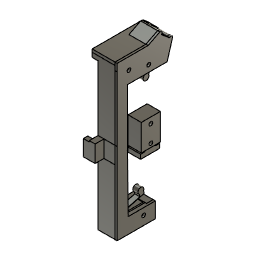
z_axis_switch v3 (Autodesk Fusion 360 design; units mm, degrees)
Autodesk Fusion 360 part; units mm, degrees
sketch "cnc " plane through (0, 0, 0) normal (1, 0, 0) x (0, 1, 0)
  line L0 (-75, 149.6) -> (-75, 72.1)
  line L1 (-75, 72.1) -> (-75, 61.1) construction
  line L2 (-75, 149.6) -> (-75, 160.6) construction
  line L3 (-75, 160.6) -> (-102, 160.6)
  line L4 (-102, 160.6) -> (-102, 61.1)
  line L5 (-102, 61.1) -> (-75, 61.1)
  line L6 (-75, 149.6) -> (-36, 149.6)
  line L7 (-75, 72.1) -> (-47, 72.1)
  line L8 (-47, 72.1) -> (-47, 61.1)
  line L9 (-47, 61.1) -> (-75, 61.1)
  line L10 (-75, 160.6) -> (-36, 160.6)
  line L11 (-36, 160.6) -> (-36, 149.6)
  line L12 (-75, 149.6) -> (-56, 149.6) construction
  line L13 (-56, 149.6) -> (-52, 149.6) construction
  line L14 (-52, 149.6) -> (-60, 149.6) construction
  line L15 (-60, 149.6) -> (-60, 67) construction
  line L16 (-60, 67) -> (-52, 67) construction
  line L17 (-52, 67) -> (-52, 149.6) construction
  line L18 (-8.6261, 128.7317) -> (-68.6261, 128.7317)
  line L19 (-68.6261, 128.7317) -> (-68.6261, 94.7317)
  line L20 (-68.6261, 94.7317) -> (-8.6261, 94.7317)
  line L21 (-8.6261, 94.7317) -> (-8.6261, 128.7317)
  dimension "d1" = 77.5
  dimension "d2" = 11
  dimension "d3" = 11
  dimension "d4" = 27
  dimension "d5" = 39
  dimension "d6" = 28
  dimension "d7" = 19
  dimension "d9" = 8
  dimension "d10" = 60
  dimension "d11" = 34
  constraint vertical L0
  constraint parallel L0 L1
  constraint vertical L2
  constraint perpendicular L2 L3
  constraint perpendicular L3 L4
  constraint perpendicular L1 L5
  constraint perpendicular L2 L6
  constraint perpendicular L1 L7
  constraint perpendicular L5 L8
  constraint perpendicular L8 L9
  constraint perpendicular L2 L10
  constraint perpendicular L6 L11
  constraint perpendicular L0 L12
  constraint parallel L6 L13
  constraint horizontal L14
  constraint vertical L15
  constraint horizontal L16
  constraint vertical L17
  constraint horizontal L18
  constraint vertical L19
  constraint horizontal L20
  constraint vertical L21
  measures "d1" distance of L0.start L0.end
  measures "d2" distance of L0.end L1.end
  measures "d3" distance of L0.start L2.end
  measures "d4" distance of L2.end L3.end
  measures "d5" distance of L0.start L6.end
  measures "d6" distance of L0.end L7.end
  measures "d7" distance of L0.start L12.end
  measures "d9" distance of L13.end L14.end
  measures "d10" distance of L18.start L18.end
  measures "d11" distance of L18.start L20.end
sketch "bracket base" plane through (0, 0, 0) normal (1, 0, 0) x (0, 1, 0)
  line L0 (-75, 111.25) -> (-88, 111.25) construction
  line L1 (-75, 111.25) -> (-77, 111.25) construction
  line L2 (-77, 111.25) -> (-77, 105.5) construction
  line L3 (-77, 105.5) -> (-80, 105.5)
  line L4 (-80, 105.5) -> (-80, 116.25)
  line L5 (-80, 116.25) -> (-77, 116.25)
  line L6 (-77, 116.25) -> (-77, 105.5)
  line L7 (-80, 117) -> (-74, 117)
  line L8 (-74, 117) -> (-74, 105.5)
  line L9 (-74, 105.5) -> (-80, 105.5)
  line L10 (-80, 105.5) -> (-80, 117)
  line L11 (-74, 161) -> (-74, 117)
  line L12 (-67, 149.9652) -> (-67, 111.25)
  line L13 (-48.0004, 72.0159) -> (-48.0011, 61.5)
  line L14 (-67, 72.0348) -> (-67, 111.25)
  line L15 (-74, 61.5) -> (-74, 105.5)
  line L16 (-74, 61.5) -> (-48.0011, 61.5)
  circle A0 centre (-56, 67.5) radius 1.25
  circle A1 centre (-66, 158) radius 1.25
  line L17 (-67, 149.9652) -> (-40.0004, 149.992)
  line L18 (-74, 161) -> (-74, 164.0222)
  line L19 (-74, 164.0222) -> (-40.0011, 163.9932)
  line L20 (-67, 72.0348) -> (-48.0004, 72.0159)
  circle A2 centre (-52.5121, 154.5) radius 1.25
  circle A3 centre (-59.5121, 154.5) radius 0.9
  circle A4 centre (-63, 67.5) radius 0.9
  line L21 (-68.5, 152) -> (-68.5, 69.9959)
  line L22 (-66, 66) -> (-66, 72)
  line L23 (-53, 72) -> (-53, 66)
  line L24 (-62.5121, 155.9825) -> (-62.5121, 149.9825)
  line L25 (-49.5121, 149.9825) -> (-49.5121, 155.9825)
  line L26 (-68.5, 152) -> (-63.083, 152)
  line L27 (-63.083, 152) -> (-63.081, 149.9691)
  line L28 (-68.5, 69.9959) -> (-66.5, 69.9959)
  line L29 (-66.5, 69.9959) -> (-66.5, 72.0343)
  line L30 (-72.5, 164.0209) -> (-72.5, 61.5)
  line L31 (-49, 152) -> (-48.998, 149.9831)
  line L32 (-49, 152) -> (-42.0325, 152.0069)
  line L33 (-57.0005, 161) -> (-57.0005, 164.0077)
  line L34 (-57.0005, 164.0077) -> (-45, 170)
  line L35 (-36.3287, 162.5038) -> (-40.0004, 149.992)
  line L36 (-40.0011, 163.9932) -> (-36.3, 163.9932)
  line L37 (-38.345, 163.1699) -> (-42.0325, 152.0069)
  line L38 (-57.0005, 161) -> (-43.8745, 167.8402)
  arc A5 (-43.8745, 167.8402) -> (-45, 170) centre (-44.7427, 168.7609) ccw
  arc A6 (-36.3287, 162.5038) -> (-38.345, 163.1699) centre (-37.3657, 162.7495) ccw
  line L39 (-43.6205, 169.3458) -> (-36.6837, 163.5684)
  line L40 (-40.0011, 161) -> (-36.77, 161)
  line L41 (-40.0011, 161) -> (-74, 161)
  line L42 (-47, 62.5) -> (-72.5, 62.5)
  line L43 (-50, 72.5) -> (-50, 62.5)
  line L44 (-52.5, 72.5) -> (-52.5, 69.9959)
  line L45 (-52.5, 69.9959) -> (-50, 69.9959)
  line L46 (-74, 166) -> (-40.1038, 166)
  line L47 (-74, 164.0222) -> (-74, 166)
  circle A7 centre (-45, 155) radius 1.25
  circle A8 centre (-43, 162) radius 1.25
  circle A9 centre (-66, 158) radius 3
  line L48 (-46.25, 155.0105) -> (-48.5, 159.5)
  line L49 (-46.524, 160.4903) -> (-43.7645, 155.19)
  arc A10 (-46.524, 160.4903) -> (-48.5, 159.5) centre (-47.5044, 159.9799) ccw
  line L50 (-40.1038, 166) -> (-39.6033, 166)
  circle A11 centre (-67.75, 66.5) radius 1.25
  dimension "d46" = 2.5
  dimension "d47" = 2.5
  dimension "d99" = 2.5
  dimension "d100" = 1.8
  dimension "d101" = 1.8
  dimension "d135" = 13
  dimension "d136" = 6
  dimension "d139" = 2.5
  dimension "d140" = 2.5
  dimension "d141" = 2.5
  constraint coincident L0 L1.end
  constraint perpendicular L0 L2
  constraint horizontal L3
  constraint vertical L4
  constraint horizontal L5
  constraint vertical L6
  constraint horizontal L7
  constraint vertical L8
  constraint horizontal L9
  constraint vertical L10
  constraint perpendicular L0 L12
  constraint coincident L16 L30.end
  constraint perpendicular L21 L26
  constraint coincident L17 L27.end
  constraint perpendicular L17 L27
  constraint perpendicular L22 L28
  constraint coincident L20 L29.end
  constraint perpendicular L28 L29
  constraint coincident L19 L30.start
  constraint coincident L17 L31.end
  constraint perpendicular L17 L31
  constraint perpendicular L31 L32
  constraint midpoint L19 L33.end
  constraint vertical L33
  constraint horizontal L36
  constraint midpoint A5 L39.start
  constraint coincident A6 L39.end
  constraint tangent A6 L39
  constraint coincident L35 L40.end
  constraint coincident L30 L42.end
  constraint perpendicular L30 L42
  constraint coincident L42 L43.end
  constraint perpendicular L42 L43
  constraint perpendicular L28 L44
  constraint coincident L43 L45.end
  constraint perpendicular L43 L45
  constraint perpendicular L46 L47
  constraint concentric A1 A9
  constraint coincident A7 L48.start
  constraint coincident A7 L49.end
  constraint tangent L49 A10
  constraint coincident L39 L50.end
  constraint parallel L46 L50
  measures "d46" diameter of A0
  measures "d47" diameter of A1
  measures "d99" diameter of A2
  measures "d100" diameter of A3
  measures "d101" diameter of A4
  measures "d135" distance of L25.start L24.end
  measures "d136" distance of L24.start L24.end
  measures "d139" diameter of A7
  measures "d140" diameter of A8
  measures "d141" diameter of A11
sketch "switches" plane through (0, 0, 0) normal (1, 0, 0) x (0, 1, 0)
  line L0 (0, 2.5) -> (0, 20)
  line L1 (-53, 66) -> (-66, 66)
  line L2 (-64.544, 66) -> (-64.544, 63)
  line L3 (-59.244, 66) -> (-59.244, 63)
  arc A0 (-51.9175, 78.8916) -> (-54.8153, 78.1152) centre (-53.3664, 78.5034) ccw
  line L4 (-51.141, 75.9939) -> (-51.0745, 75.7529)
  line L5 (-55, 65.5) -> (-54.514, 66)
  line L6 (-54.514, 63) -> (-54.514, 66)
  line L7 (-66, 66) -> (-66, 72)
  circle A1 centre (-53.3664, 78.5034) radius 2
  circle A2 centre (-56, 67.5) radius 0.9
  line L8 (-54.014, 66) -> (-54.014, 63)
  line L9 (-59.244, 63) -> (-59.744, 63)
  line L10 (-65.0804, 72) -> (-65.1451, 72.2415)
  line L11 (-64, 65.5) -> (-62, 65.5)
  line L12 (-57, 65.5) -> (-55, 65.5)
  line L13 (-54.0388, 75.2174) -> (-54.8153, 78.1152)
  line L14 (-65.044, 63) -> (-65.044, 66)
  line L15 (-66, 72) -> (-53, 72)
  circle A3 centre (-63, 67.5) radius 0.9
  line L16 (-51.141, 75.9939) -> (-51.9175, 78.8916)
  line L17 (-64, 65.5) -> (-64.5144, 66)
  line L18 (-51.141, 75.9939) -> (-54.0388, 75.2174)
  line L19 (-65.1451, 72.2415) -> (-51.141, 75.9939)
  line L20 (-65.0804, 72) -> (-51.0745, 75.7529)
  line L21 (-59.744, 66) -> (-59.244, 66)
  line L22 (-54.514, 66) -> (-54.014, 66)
  line L23 (-65.044, 66) -> (-64.544, 66)
  line L24 (-59.744, 63) -> (-59.744, 66)
  line L25 (-64.544, 63) -> (-65.044, 63)
  line L26 (-53, 72) -> (-53, 66)
  line L27 (-62, 65.5) -> (-61.514, 66)
  line L28 (-54.014, 63) -> (-54.514, 63)
  line L29 (-57, 65.5) -> (-57.5144, 66)
  line L30 (-47.6531, 145.9886) -> (-50.5509, 146.7651)
  line L31 (-61.6572, 149.741) -> (-47.6531, 145.9886)
  line L32 (-51.026, 155.9825) -> (-50.526, 155.9825)
  line L33 (-60.5121, 156.4825) -> (-58.5121, 156.4825)
  line L34 (-50.5509, 146.7651) -> (-51.3273, 143.8673)
  line L35 (-49.5121, 149.9825) -> (-49.5121, 155.9825)
  circle A4 centre (-49.8784, 143.4791) radius 2
  line L36 (-51.026, 158.9825) -> (-51.026, 155.9825)
  line L37 (-61.056, 155.9825) -> (-61.056, 158.9825)
  line L38 (-53.5121, 156.4825) -> (-54.0264, 155.9825)
  line L39 (-50.526, 158.9825) -> (-51.026, 158.9825)
  line L40 (-61.5925, 149.9825) -> (-47.5865, 146.2296)
  line L41 (-56.256, 158.9825) -> (-56.256, 155.9825)
  line L42 (-61.5925, 149.9825) -> (-61.6572, 149.741)
  line L43 (-62.5121, 155.9825) -> (-62.5121, 149.9825)
  line L44 (-53.5121, 156.4825) -> (-51.5121, 156.4825)
  line L45 (-47.6531, 145.9886) -> (-47.5865, 146.2296)
  line L46 (-51.5121, 156.4825) -> (-51.026, 155.9825)
  line L47 (-56.256, 155.9825) -> (-55.756, 155.9825)
  line L48 (-61.056, 158.9825) -> (-61.556, 158.9825)
  circle A5 centre (-52.5121, 154.4825) radius 0.9
  arc A6 (-51.3273, 143.8673) -> (-48.4296, 143.0909) centre (-49.8784, 143.4791) ccw
  circle A7 centre (-59.5121, 154.4825) radius 0.9
  line L49 (-61.556, 155.9825) -> (-61.056, 155.9825)
  line L50 (-58.5121, 156.4825) -> (-58.026, 155.9825)
  line L51 (-62.5121, 149.9825) -> (-49.5121, 149.9825)
  line L52 (-55.756, 155.9825) -> (-55.756, 158.9825)
  line L53 (-50.526, 155.9825) -> (-50.526, 158.9825)
  line L54 (-47.6531, 145.9886) -> (-48.4296, 143.0909)
  line L55 (-60.5121, 156.4825) -> (-61.0264, 155.9825)
  line L56 (-49.5121, 155.9825) -> (-62.5121, 155.9825)
  line L57 (-55.756, 158.9825) -> (-56.256, 158.9825)
  line L58 (-61.556, 158.9825) -> (-61.556, 155.9825)
  line L59 (-57.6, 101) -> (-44.6, 101)
  line L60 (-57.6, 123) -> (-44.6, 123)
  line L61 (-57.6, 123) -> (-57.6, 105)
  line L62 (-57.6, 105) -> (-44.6, 105)
  line L63 (-44.6, 105) -> (-44.6, 123)
  circle A8 centre (-51.1, 119) radius 1.25
  circle A9 centre (-51.1, 107.5) radius 1.25
  line L64 (-44.6, 101) -> (-44.6, 104)
  line L65 (-44.6, 104) -> (-47.6, 104)
  line L66 (-47.6, 104) -> (-47.6, 121)
  line L67 (-47.6, 121) -> (-54.6, 121)
  line L68 (-54.6, 121) -> (-54.6, 105)
  line L69 (-57.6, 101) -> (-57.6, 104)
  line L70 (-57.6, 104) -> (-54.6, 104)
  line L71 (-54.6, 104) -> (-54.6, 105)
  line L72 (-52.3542, 105) -> (-52.3542, 121)
  line L73 (-49.8734, 105) -> (-49.8734, 121)
  line L74 (-49.8784, 143.4791) -> (-49.8784, 65) construction
  line L75 (-53.3664, 78.5034) -> (-53.3664, 167.4772) construction
  dimension "d74" = 13
  dimension "d75" = 6
  dimension "d76" = 1.8
  dimension "d77" = 1.8
  dimension "d78" = 0.5
  dimension "d79" = 3
  dimension "d80" = 0.5
  dimension "d81" = 3
  dimension "d82" = 0.5
  dimension "d83" = 3
  dimension "d85" = 14.5
  dimension "d86" = 0.25
  dimension "d87" = 3
  dimension "d88" = 3
  dimension "d89" = 3
  dimension "d90" = 4
  dimension "d91" = 2.5
  dimension "d92" = 2.5
  dimension "d97" = 1.8
  dimension "d98" = 1.8
  constraint coincident L50.end L56
  constraint coincident L55.end L56
  constraint perpendicular L50 L55
  constraint parallel L44 L56
  constraint coincident L32.start L56
  constraint parallel L46 L50
  constraint coincident L38.end L56
  constraint perpendicular L38 L50
  constraint coincident L40.start L51
  constraint perpendicular L40 L42
  constraint perpendicular L31 L42
  constraint perpendicular L31 L54
  constraint perpendicular L30 L54
  constraint perpendicular L31 L34
  constraint tangent A6 L54
  constraint concentric A4 A6
  constraint horizontal L59
  constraint horizontal L60
  constraint perpendicular L60 L61
  constraint perpendicular L61 L62
  constraint perpendicular L60 L63
  constraint perpendicular L59 L64
  constraint perpendicular L64 L65
  constraint perpendicular L60 L66
  constraint perpendicular L66 L67
  constraint coincident L62 L68.end
  constraint perpendicular L60 L68
  constraint perpendicular L59 L69
  constraint perpendicular L69 L70
  constraint perpendicular L62 L71
  constraint coincident L62 L72.start
  constraint coincident L67 L72.end
  constraint perpendicular L67 L72
  constraint coincident L62 L73.start
  constraint coincident L67 L73.end
  constraint perpendicular L67 L73
  constraint coincident A4.centre A6.centre
  constraint perpendicular L59 L74
  constraint coincident A0.centre A1.centre
  constraint perpendicular L56 L75
  measures "d74" distance of L43.end L35.start
  measures "d75" distance of L43.start L43.end
  measures "d76" diameter of A7
  measures "d77" diameter of A5
  measures "d78" distance of L32.end L32.start
  measures "d79" distance of L36.start L32.start
  measures "d80" distance of L47.end L41.end
  measures "d81" distance of L41.start L41.end
  measures "d82" distance of L49.start L37.start
  measures "d83" distance of L49.start L48.end
  measures "d85" distance of L40.end L40.start
  measures "d86" distance of L31.start L40.start
  measures "d87" distance of A6.end L30.start
  measures "d88" distance of L30.end L30.start
  measures "d89" distance of L30.end L34.end
  measures "d90" diameter of A4
  measures "d91" diameter of A8
  measures "d92" diameter of A9
  measures "d97" diameter of A3
  measures "d98" diameter of A2
extrude "Extrude8" add sketch "bracket base" against normal blind 8 contours L3 L4 L5 L6 L9 L10 | L18 L19 L30 L41 | L19 L34 L46 L47 | L19 L30 L33 L41 | L19 L34 L38 L46 | L19 L33 L38 | L19 L36 L37 L38 A6 L39 L40 L41 A8 A10 | L19 L36 L38 L39 L46 L50 | L41 A8 | L35 L37 A6 L40 picked at (-42.8725, 161.8242) makes body 1 at (-2.6667, -80, 109.0833) makes body 2 at (-2.6667, -62.5344, 166)
extrude "Extrude12" add sketch "bracket base" against normal blind 4 contours L5 L6 L7 L8 L9 L10 | L8 L11 L15 L16 L30 L41 | L18 L19 L30 L41 | L13 L16 L30 L42 | L19 L34 L46 L47 | A9 | L17 L20 L21 L26 L27 L28 L29 L30 L31 L32 L37 L40 L41 L42 L43 L44 L45 A7 A8 L48 L49 A10 | L19 L30 L33 L41 | L13 L20 L42 L43 | L19 L34 L38 L46 | L19 L33 L38 | L34 L38 A5 L46 | L19 L36 L37 L38 A6 L39 L40 L41 A8 A10 | L20 L43 L44 L45 | L19 L36 L38 L39 L46 L50 | L38 A5 L39 L46 L50 | L41 A10 | L41 A7 L48 L49 A10 | L41 A8 | L41 A8 | A7 L49 | L12 L14 L17 L20 L21 L26 L27 L28 L29 | L35 L37 A6 L40 | A7 L49 | L17 L31 L32 L35 L37 L40 | A11 bodies 2 1
extrude "Extrude10" add sketch "switches" along normal blind 5.5 separate body contours L1 L7 L15 L21 L22 L23 L26 | L32 L35 L43 L47 L49 L51 L56 makes body 3 at (0, -54.9954, 151.2227) makes body 4 at (0, -58.4833, 70.7598)
extrude "Extrude11" add sketch "switches" along normal blind 4.5 and the other way blind -1 contours L4 L10 L18 L19 L20 | L1 L6 L8 L22 L28 | L1 L5 L12 L29 | L1 L3 L9 L21 L24 | A1 L13 L16 L18 L19 | A0 A1 L13 L16 | A0 A1 L13 L16 | L1 L2 L14 L23 L25 | L1 L11 L17 L27 | L30 L31 L34 A4 L54 | L30 L31 L40 L42 L45 | L34 A4 A6 L54 | L34 A4 A6 L54 | L37 L48 L49 L56 L58 | L32 L36 L39 L53 L56 | L38 L44 L46 L56 | L33 L50 L55 L56 | L41 L47 L52 L56 L57 bodies 3 4
extrude "Extrude16" add sketch "switches" along normal blind 9 and the other way blind -7 separate body contours L62 L67 L68 L72 | L60 L61 L62 L63 L66 L67 L68 | L62 A8 A9 L66 L67 L73 | L62 A8 A9 L67 L72 L73 makes body 5
extrude "Extrude17" add sketch "switches" along normal blind 7 contours L60 L61 L62 L63 L66 L67 L68 bodies 5
extrude "Extrude18" add sketch "switches" along normal blind 7 separate body contours L62 L67 L68 L72 | L62 A8 A9 L66 L67 L73 | A9 L73 | A8 L73 picked at (-49.8691, 107.4463) picked at (-49.8691, 118.9463) makes body 6 at (2.3333, -54.6, 115.6667) makes body 7 at (2.3333, -47.6, 110.3333)
extrude "Extrude19" add sketch "switches" along normal blind 8.5 contours L59 L62 L64 L65 L66 L69 L70 L71 bodies 6 7
move_face "OffsetFaces3" offset -0.4 3 faces at (2.3333, -49.9333, 121) (2.3333, -47.6, 110.3333) (2.3333, -54.6, 115.6667) on bodies 5
move_face "OffsetFaces4" offset 0.1 1 faces at (0, -49.9333, 102) on bodies 6
extrude "Extrude20" add sketch "bracket base" along normal blind 7.5 contours L8 L11 L15 L16 L30 L41 | L18 L19 L30 L41 | L13 L16 L30 L42 | L19 L34 L46 L47 | A9 | L13 L20 L42 L43 | L19 L34 L38 L46 | L34 L38 A5 L46 | L20 L43 L44 L45 | L41 A10 | L41 A7 L48 L49 A10 | L41 A8 | L41 A8 | A7 L49 | L12 L14 L17 L20 L21 L26 L27 L28 L29 | L35 L37 A6 L40 | A7 L49 | L17 L31 L32 L35 L37 L40 | A11 bodies 2
sketch "cover" plane through (7.5, 0, 0) normal (1, 0, 0) x (0, 1, 0)
  line L0 (-74, 164.0222) -> (-74, 117)
  line L1 (-74, 117) -> (-74, 105.5)
  line L2 (-74, 105.5) -> (-74, 61.5)
  line L3 (-74, 61.5) -> (-48.0011, 61.5)
  line L4 (-48.0011, 61.5) -> (-48.0004, 72.0159)
  line L5 (-48.0004, 72.0159) -> (-52.5, 72.0204)
  line L6 (-52.5, 72.0204) -> (-52.5, 69.9959)
  line L7 (-51.2384, 164.0028) -> (-43.8745, 167.8402)
  arc A0 (-43.8745, 167.8402) -> (-45, 170) centre (-44.7427, 168.7609) ccw
  line L8 (-45, 170) -> (-53.0106, 166)
  line L9 (-53.0106, 166) -> (-74, 166)
  line L10 (-74, 166) -> (-74, 164.0222)
  line L11 (-57.0005, 164.0077) -> (-45, 170)
  line L12 (-74, 166) -> (-40.1038, 166)
  arc A1 (-36.3287, 162.5038) -> (-38.345, 163.1699) centre (-37.3657, 162.7495) ccw
  line L13 (-36.3287, 162.5038) -> (-40.0004, 149.992)
  arc A2 (-43.8745, 167.8402) -> (-45, 170) centre (-44.7427, 168.7609) ccw
  line L14 (-49, 152) -> (-48.998, 149.9831)
  line L15 (-67, 149.9652) -> (-40.0004, 149.992)
  line L16 (-74, 161) -> (-74, 117)
  line L17 (-74, 61.5) -> (-48.0011, 61.5)
  line L18 (-67, 72.0348) -> (-67, 111.25)
  line L19 (-66.5, 69.9959) -> (-66.5, 72.0343)
  line L20 (-52.5, 72.5) -> (-52.5, 69.9959)
  circle A3 centre (-66, 158) radius 1.25
  circle A4 centre (-52.5121, 154.5) radius 1.25
  circle A5 centre (-56, 67.5) radius 1.25
  line L21 (-63.083, 152) -> (-49, 152)
  line L22 (-63.083, 152) -> (-63.081, 149.9691)
  line L23 (-66.5, 72.0343) -> (-52.5, 72.0204)
  line L24 (-66.5, 69.9959) -> (-52.5, 69.9959)
  line L25 (-43.8745, 167.8402) -> (-38.345, 163.1699)
  line L26 (-67, 149.9652) -> (-67, 111.25)
  line L27 (-74, 166) -> (-74, 161)
  line L28 (-48.0011, 61.5) -> (-48.0004, 72.0159)
  line L29 (-48.0004, 72.0159) -> (-52.5, 72.0204)
  line L30 (-74, 61.5) -> (-74, 117)
  line L31 (-74, 161) -> (-74, 117)
  line L32 (-74, 61.5) -> (-48.0011, 61.5)
  line L33 (-66.5, 72.0343) -> (-67, 111.25)
  line L34 (-72.5, 62.5) -> (-70.5, 62.5)
  line L35 (-70.5, 62.5) -> (-70.5, 64.5)
  line L36 (-70.5, 64.5) -> (-72.5, 64.5)
  line L37 (-72.5, 64.5) -> (-72.5, 62.5)
  line L38 (-72.5, 164) -> (-70.5, 164)
  line L39 (-70.5, 164) -> (-70.5, 162)
  line L40 (-70.5, 162) -> (-72.5, 162)
  line L41 (-72.5, 162) -> (-72.5, 164)
  constraint coincident L14.start L21.end
  constraint coincident L15 L22.end
  constraint perpendicular L15 L22
  constraint coincident L19.end L23.start
  constraint coincident L5.end L6.start
  constraint coincident A1.end L25.end
  constraint coincident L15.start L26.start
  constraint coincident L18.end L26.end
  constraint coincident L9.end L10.start
  constraint coincident L16.start L27.end
  constraint coincident L3.end L4.start
  constraint coincident L4.end L5.start
  constraint coincident L2.end L3.start
  constraint coincident L0.end L1.start
  constraint horizontal L34
  constraint vertical L35
  constraint horizontal L36
  constraint vertical L37
  constraint horizontal L38
  constraint vertical L39
  constraint horizontal L40
  constraint vertical L41
extrude "Extrude21" add sketch "cover" against normal blind 1 separate body contours L6 L19 L20 L23 L24 | L14 L15 L21 L22 | L34 L35 L36 L37 | L38 L39 L40 L41 makes body 8 at (7.5, -61.8333, 71.3502) makes body 9 at (7.5, -58.388, 151.323) makes body 10 at (7.5, -71.8333, 63.8333) makes body 11 at (7.5, -71.8333, 163.3333)
extrude "Extrude22" add sketch "cover" along normal blind 1.5 contours L0 L1 L2 L3 L4 L5 L6 L9 L10 L12 A1 L13 L14 L15 L16 L17 L19 L20 L21 L22 L24 L25 L26 L27 L28 L29 L30 L31 L32 L33 | L7 A0 L8 L11 L12 A2 | L7 L12 L25 | L6 L19 L20 L23 L24 | L14 L15 L21 L22 | L34 L35 L36 L37 | L38 L39 L40 L41 bodies 9 10 8 11
move_face "OffsetFaces5" offset -0.15 4 faces at (7.1667, -72.5, 162.6667) (7.1667, -72.5, 63.8333) (7.1667, -71.8333, 62.5) (7.1667, -71.8333, 164) on bodies 9
named bodies: "z_axis_switch2_base", "top switch", "bottom switch", "z_axis_stop_top", "z_axis_stop_bottom", "z_axis_switch2_cover"
